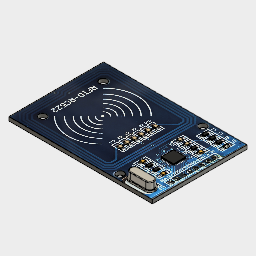
gaming node v3 (Autodesk Fusion 360 archive; units mm, degrees)
design "_RFID-RC522.cd1ec80f-b667-4655-b6b3-a21b5d1b7a74"
Autodesk Fusion 360 part; units mm, degrees
sketch "Sketch1" plane through (0, 0, 0) normal (0, 1, 0) x (1, 0, 0) in component "Base"
  line L0 (0, 0) -> (60, 0)
  line L1 (60, 0) -> (60, -39.6)
  line L2 (60, -39.6) -> (0, -39.6)
  line L3 (0, -39.6) -> (0, 0)
  circle A0 centre (7.05, -32.45) radius 1.55
  line L4 (5.5, -34) -> (0, -34) construction
  line L5 (5.5, -34) -> (5.5, -39.6) construction
  circle A1 centre (7.05, -7.15) radius 1.55
  line L6 (5.5, 0) -> (5.5, -5.6) construction
  line L7 (5.5, -5.6) -> (0, -5.6) construction
  line L8 (0, -1.0831) -> (42.4499, -1) construction
  line L9 (42.4499, -1) -> (42.4499, 0) construction
  circle A2 centre (43.9999, -2.547) radius 1.55
  line L10 (0, -38.6) -> (42.45, -38.6) construction
  line L11 (42.45, -38.6) -> (42.45, -39.6) construction
  circle A3 centre (44, -37.05) radius 1.55
  line L12 (49.05, -33.9) -> (55.45, -33.9)
  line L13 (57.6, -36.05) -> (57.6, -36.15)
  line L14 (55.45, -38.3) -> (49.05, -38.3)
  line L15 (46.9, -36.15) -> (46.9, -36.05)
  arc A4 (49.05, -33.9) -> (46.9, -36.05) centre (49.05, -36.05) ccw
  arc A5 (46.9, -36.15) -> (49.05, -38.3) centre (49.05, -36.15) ccw
  arc A6 (57.6, -36.05) -> (55.45, -33.9) centre (55.45, -36.05) ccw
  arc A7 (55.45, -38.3) -> (57.6, -36.15) centre (55.45, -36.15) ccw
  line L16 (55.45, -37.85) -> (49.05, -37.85)
  arc A8 (47.35, -36.15) -> (49.05, -37.85) centre (49.05, -36.15) ccw
  line L17 (47.35, -36.15) -> (47.35, -36.05)
  arc A9 (49.05, -34.35) -> (47.35, -36.05) centre (49.05, -36.05) ccw
  line L18 (49.05, -34.35) -> (55.45, -34.35)
  arc A10 (57.15, -36.05) -> (55.45, -34.35) centre (55.45, -36.05) ccw
  line L19 (57.15, -36.05) -> (57.15, -36.15)
  arc A11 (55.45, -37.85) -> (57.15, -36.15) centre (55.45, -36.15) ccw
  line L20 (46.9, -38.3) -> (46.9, -39.6) construction
  line L21 (57.6, -33.9) -> (60, -33.9) construction
  line L22 (58, -39.6) -> (58, -29.2) construction
  line L23 (58, -29.2) -> (60, -29.2) construction
  circle A12 centre (58, -29.2) radius 0.525
  circle A13 centre (58, -26.7) radius 0.525
  circle A14 centre (58, -24.2) radius 0.525
  circle A15 centre (58, -21.7) radius 0.525
  circle A16 centre (58, -19.2) radius 0.525
  circle A17 centre (58, -16.7) radius 0.525
  circle A18 centre (58, -14.2) radius 0.525
  circle A19 centre (58, -11.7) radius 0.525
  point P0 (46.9, -33.9)
  point P1 (57.6, -33.9)
  point P2 (46.9, -38.3)
  dimension "d1" = 60
  dimension "d2" = 39.6
  dimension "d5" = 3.1
  dimension "d8" = 5.6
  dimension "d9" = 5.5
  dimension "d10" = 3.1
  dimension "d11" = 5.6
  dimension "d12" = 5.5
  dimension "d13" = 42.45
  dimension "d14" = 1
  dimension "d15" = 3.1
  dimension "d16" = 42.45
  dimension "d17" = 1
  dimension "d18" = 3.1
  dimension "d19" = 10.7
  dimension "d20" = 4.4
  dimension "d23" = 0.45
  dimension "d24" = 2.15
  dimension "d25" = 2.4
  dimension "d26" = 1.3
  dimension "d27" = 10.4
  dimension "d28" = 2
  dimension "d29" = 1.05
  dimension "d32" = 0
  dimension "d33" = 2.5
  measures "d1" distance of L0.start L0.end
  measures "d2" distance of L0.start L2.end
  measures "d5" diameter of A0
  measures "d8" distance of L4.start L5.end
  measures "d9" distance of L4.start L4.end
  measures "d10" diameter of A1
  measures "d11" distance of L6.start L6.end
  measures "d12" distance of L6.end L7.end
  measures "d13" distance of L8.start L8.end
  measures "d14" distance of L8.end L9.end
  measures "d15" diameter of A2
  measures "d16" distance of L10.start L10.end
  measures "d17" distance of L10.end L11.end
  measures "d18" diameter of A3
  measures "d19" distance of P0 P1
  measures "d20" distance of P0 P2
  measures "d24" radius of A4
  measures "d25" distance of P1 L21.end
  measures "d26" distance of P2 L20.end
  measures "d27" distance of L22.start L22.end
  measures "d28" distance of L22.end L23.end
  measures "d29" diameter of A12
extrude "Extrude1" add sketch "Sketch1" against normal blind 1.6 contours L0 L1 L2 L3 | L12 L13 L14 L15 A4 A5 A6 A7 | L16 A8 L17 A9 L18 A10 L19 A11 makes body 1 in component "Base"
extrude "Extrude2" add sketch "Sketch1" along normal blind 0.7 separate body contours L12 L13 L14 L15 A4 A5 A6 A7 | L16 A8 L17 A9 L18 A10 L19 A11 makes body 2 in component "Base"
extrude "Extrude3" add sketch "Sketch1" along normal blind 3.55 separate body contours L16 A8 L17 A9 L18 A10 L19 A11 makes body 3 in component "Base"
fillet "Fillet1" radius 0.25 8 edges at (47.35, 3.55, 36.1) (47.8479, 3.55, 37.3521) (52.25, 3.55, 37.85) (56.6521, 3.55, 37.3521) (57.15, 3.55, 36.1) (56.6521, 3.55, 34.8479) (52.25, 3.55, 34.35) (47.8479, 3.55, 34.8479) on bodies 3 in component "Base"
combine "Combine1" operation add target body 2 tool bodies 3 in component "Base"
sketch "Sketch2" plane through (0, 0, 0) normal (0, 1, 0) x (1, 0, 0) in component "Base"
  line L0 (47.0522, -4.3477) -> (48.2693, -4.3477)
  line L1 (48.2693, -4.3477) -> (48.2693, -6.0785)
  line L2 (48.2693, -6.0785) -> (47.0522, -6.0785)
  line L3 (47.0522, -6.0785) -> (47.0522, -4.3477)
  line L4 (49.9732, -4.226) -> (51.1904, -4.226)
  line L5 (51.1904, -4.226) -> (51.1904, -5.9568)
  line L6 (51.1904, -5.9568) -> (49.9732, -5.9568)
  line L7 (49.9732, -5.9568) -> (49.9732, -4.226)
  line L8 (52.7686, -4.3029) -> (53.9858, -4.3029)
  line L9 (53.9858, -4.3029) -> (53.9858, -6.0337)
  line L10 (53.9858, -6.0337) -> (52.7686, -6.0337)
  line L11 (52.7686, -6.0337) -> (52.7686, -4.3029)
  line L12 (55.7501, -4.3253) -> (56.9673, -4.3253)
  line L13 (56.9673, -4.3253) -> (56.9673, -6.0561)
  line L14 (56.9673, -6.0561) -> (55.7501, -6.0561)
  line L15 (55.7501, -6.0561) -> (55.7501, -4.3253)
  line L16 (43.8016, -11.8351) -> (45.0188, -11.8351)
  line L17 (45.0188, -11.8351) -> (45.0188, -13.0727)
  line L18 (45.0188, -13.0727) -> (43.8016, -13.0727)
  line L19 (43.8016, -13.0727) -> (43.8016, -11.8351)
  line L20 (46.8056, -11.8576) -> (48.0227, -11.8576)
  line L21 (48.0227, -11.8576) -> (48.0227, -13.0951)
  line L22 (48.0227, -13.0951) -> (46.8056, -13.0951)
  line L23 (46.8056, -13.0951) -> (46.8056, -11.8576)
  line L24 (43.8016, -11.8351) -> (45.0188, -11.8351)
  line L25 (45.0188, -11.8351) -> (45.0188, -13.0727)
  line L26 (45.0188, -13.0727) -> (43.8016, -13.0727)
  line L27 (43.8016, -13.0727) -> (43.8016, -11.8351)
  line L28 (49.675, -11.7006) -> (50.8922, -11.7006)
  line L29 (50.8922, -11.7006) -> (50.8922, -13.4314)
  line L30 (50.8922, -13.4314) -> (49.675, -13.4314)
  line L31 (49.675, -13.4314) -> (49.675, -11.7006)
  line L32 (52.5668, -11.9024) -> (53.784, -11.9024)
  line L33 (53.784, -11.9024) -> (53.784, -13.14)
  line L34 (53.784, -13.14) -> (52.5668, -13.14)
  line L35 (52.5668, -13.14) -> (52.5668, -11.9024)
  line L36 (46.8596, -17.6793) -> (52.06, -17.6793)
  line L37 (52.06, -17.6793) -> (52.06, -22.8023)
  line L38 (52.06, -22.8023) -> (46.8596, -22.8023)
  line L39 (46.8596, -22.8023) -> (46.8596, -17.6793)
  line L40 (33.7509, -12.0901) -> (35.1413, -12.0901)
  line L41 (35.1413, -12.0901) -> (35.1413, -13.3759)
  line L42 (35.1413, -13.3759) -> (33.7509, -13.3759)
  line L43 (33.7509, -13.3759) -> (33.7509, -12.0901)
  line L44 (33.736, -15.0653) -> (35.1264, -15.0653)
  line L45 (33.736, -16.3511) -> (33.736, -15.0653)
  line L46 (35.1264, -15.0653) -> (35.1264, -16.3511)
  line L47 (35.1264, -16.3511) -> (33.736, -16.3511)
  line L48 (33.6911, -17.9209) -> (35.0815, -17.9209)
  line L49 (33.6911, -19.2067) -> (33.6911, -17.9209)
  line L50 (35.0815, -17.9209) -> (35.0815, -19.2067)
  line L51 (35.0815, -19.2067) -> (33.6911, -19.2067)
  line L52 (33.6691, -20.8381) -> (35.0596, -20.8381)
  line L53 (33.6691, -22.1239) -> (33.6691, -20.8381)
  line L54 (35.0596, -20.8381) -> (35.0596, -22.1239)
  line L55 (35.0596, -22.1239) -> (33.6691, -22.1239)
  line L56 (33.7108, -23.8497) -> (35.1012, -23.8497)
  line L57 (33.7108, -25.1354) -> (33.7108, -23.8497)
  line L58 (35.1012, -23.8497) -> (35.1012, -25.1354)
  line L59 (35.1012, -25.1354) -> (33.7108, -25.1354)
  line L60 (33.7803, -26.782) -> (35.1708, -26.782)
  line L61 (33.7803, -28.0678) -> (33.7803, -26.782)
  line L62 (35.1708, -26.782) -> (35.1708, -28.0678)
  line L63 (35.1708, -28.0678) -> (33.7803, -28.0678)
  line L64 (43.9054, -27.4668) -> (45.1225, -27.4668)
  line L65 (45.1225, -27.4668) -> (45.1225, -28.7044)
  line L66 (45.1225, -28.7044) -> (43.9054, -28.7044)
  line L67 (43.9054, -28.7044) -> (43.9054, -27.4668)
  line L68 (43.8016, -11.8351) -> (45.0188, -11.8351)
  line L69 (45.0188, -11.8351) -> (45.0188, -13.0727)
  line L70 (45.0188, -13.0727) -> (43.8016, -13.0727)
  line L71 (43.8016, -13.0727) -> (43.8016, -11.8351)
  line L72 (52.5824, -27.5841) -> (53.7996, -27.5841)
  line L73 (53.7996, -27.5841) -> (53.7996, -28.8217)
  line L74 (53.7996, -28.8217) -> (52.5824, -28.8217)
  line L75 (52.5824, -28.8217) -> (52.5824, -27.5841)
  line L76 (46.643, -27.2525) -> (47.8602, -27.2525)
  line L77 (47.8602, -27.2525) -> (47.8602, -28.9833)
  line L78 (47.8602, -28.9833) -> (46.643, -28.9833)
  line L79 (46.643, -28.9833) -> (46.643, -27.2525)
  line L80 (49.5422, -27.2928) -> (50.7594, -27.2928)
  line L81 (50.7594, -27.2928) -> (50.7594, -29.0236)
  line L82 (50.7594, -29.0236) -> (49.5422, -29.0236)
  line L83 (49.5422, -29.0236) -> (49.5422, -27.2928)
extrude "Extrude4" add sketch "Sketch2" along normal blind 0.5 separate body makes body 4 at (49.948, 0, 28.4466) makes body 5 at (50.0807, 0, 12.2776) makes body 6 at (34.6378, 0, 24.7069) makes body 7 at (34.2144, 0, 12.5187) makes body 8 at (50.379, 0, 5.3799) makes body 9 at (56.1558, 0, 4.9022) makes body 10 at (34.1326, 0, 21.2667) makes body 11 at (47.2113, 0, 12.6826) makes body 12 at (47.0487, 0, 28.4064) makes body 13 at (52.9881, 0, 27.9966) makes body 14 at (52.9726, 0, 12.3149) makes body 15 at (34.2438, 0, 27.2106) makes body 16 at (34.1994, 0, 15.4939) makes body 17 at (47.8636, 0, 5.5016) makes body 18 at (53.1743, 0, 4.8798) makes body 19 at (34.1546, 0, 18.3495) makes body 20 at (44.6131, 0, 12.2477) makes body 21 at (44.3111, 0, 28.2919) makes body 22 at (48.5931, 0, 19.3869) in component "Base"
component "Base" placed x (1, 0, 0) y (0, 1, 0) z (0, 0, 1) at (0, 0, 0)
component "Pins" placed x (1, 0, 0) y (0, 1, 0) z (0, 0, 1) at (0, 0, 0)
equation "d39 = 5.15 mm - 1.6 mm"
named bodies: "base", "Clock"
